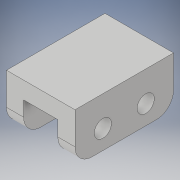
# Autodesk Inventor part: Y_Slider_Part_mit_Schrittmotor
Saved by Autodesk Inventor 2019 (Build 230136000, 136)
## iProperties
Created: 2018-08-19
Part Number: Y_Slider_Part_mit_Schrittmotor
Material: Generic
Document SubType Name: Modeling
Designer: Julia
Density: 1 g/cm^3
Appearance: Default
Author: Julia
Autodesk Inventor part; units mm, degrees
ref_plane "YZ Plane" through (0, 0, 0) normal (1, 0, 0) x (0, 1, 0)
ref_plane "XZ Plane" through (0, 0, 0) normal (0, 1, 0) x (-1, 0, 0)
ref_plane "XY Plane" through (0, 0, 0) normal (0, 0, 1) x (1, 0, 0)
sketch "Sketch1" plane through (0, 0, 0) normal (0, 1, 0) x (-1, 0, 0)
  line L0 (40, 57.5) -> (-40, 57.5)
  line L1 (-40, 57.5) -> (-40, -57.5)
  line L2 (-40, -57.5) -> (40, -57.5)
  line L3 (40, -57.5) -> (40, 57.5)
  point P0 (0, 0)
  point P1 (40, 0)
  point P2 (0, 57.5)
  dimension "d0" = 115
  dimension "d1" = 80
  constraints: 8 end point, 2 midpoint, 2 parallel, 1 horizontal, 1 horizontal alignment, 1 perpendicular, 1 vertical alignment
  measures "d0" distance of L2.end L0.start
  measures "d1" distance of L1.end L2.end
extrude "Extrusion1" add sketch "Sketch1" along normal blind 20
sketch "Sketch12" plane through (0, 0, 0) normal (0, -1, 0) x (1, 0, 0)
  line L0 (-40, 57.5) -> (-20, 57.5)
  line L1 (-20, 57.5) -> (-20, -57.5)
  line L2 (-20, -57.5) -> (-40, -57.5)
  line L3 (-40, -57.5) -> (-40, 57.5)
  line L4 (-40, -57.5) -> (-40, 57.5) projected
  line L5 (0, 100.8809) -> (0, -116.5773) construction
  line L6 (40, 57.5) -> (20, 57.5)
  line L7 (20, 57.5) -> (20, -57.5)
  line L8 (20, -57.5) -> (40, -57.5)
  line L9 (40, -57.5) -> (40, 57.5)
  point P0 (0, 0)
  point P1 (-40, 0)
  point P2 (0, 0)
  point P3 (-20, 0)
  dimension "d56" = 20
  dimension "d57" = 115
  constraints: 18 end point, 4 symmetric about line, 2 horizontal alignment, 2 midpoint, 2 parallel, 2 vertical, 1 collinear, 1 horizontal, 1 perpendicular
  measures "d56" distance of L0.start L0.end
  measures "d57" distance between parallel lines of L2 L0
extrude "Extrusion11" add sketch "Sketch12" along normal blind 37.5
sketch "Sketch13" plane through (-40, 0, 57.5) normal (-1, 0, 0) x (0, 0, 1)
  line L0 (0, 0) -> (-115, 0) projected
  point P0 (-57.5, 0)
  point P1 (-32.5, -15)
  point P2 (-82.5, -15)
  point P3 (-57.5, -15)
  point P4 (-57.5, 0)
  dimension "d129" = 25
  dimension "d130" = 25
  dimension "d131" = 15
  constraints: 2 horizontal alignment, 1 midpoint, 1 vertical alignment
  measures "d129" horizontal distance of point (-57.5, 0) point (-82.5, -15)
  measures "d130" horizontal distance of point (-32.5, -15) point (-57.5, 0)
  measures "d131" distance of point (-57.5, 0) point (-57.5, -15)
hole "Hole2" at (-40, -15, 25) at (-40, -15, -25) direction (1, 0, 0) diameter 20 end through all
fillet "Fillet19" radius 20 4 edges at (-30, -37.5, -57.5) (30, -37.5, -57.5) (30, -37.5, 57.5) (-30, -37.5, 57.5)
body "Solid1"
